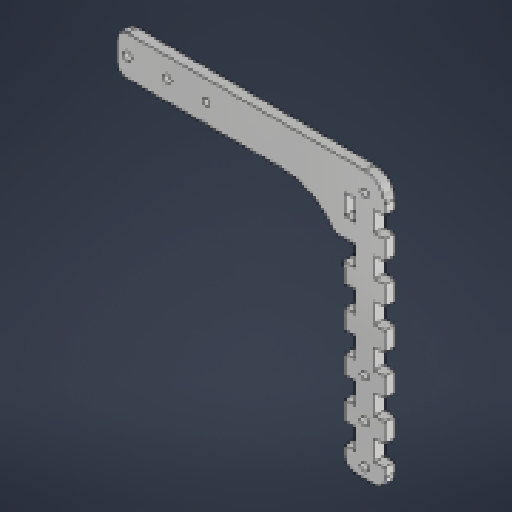
# Autodesk Inventor part: PLATE,CLAMP,MK4i,Swerve,CUSTOM,FRC2026
Saved by Autodesk Inventor 2026.1 (Build 301233020, 233B)
## iProperties
Created: 2021-12-05
Part Number: PLATE,CLAMP,MK4i,Swerve,CUSTOM,FRC2026
Material: Aluminum 7075
Document SubType Name: Modeling
Designer: dave.simone
Density: 2.81 g/cm^3
Appearance: Aluminum - Polished
Mass: 126.09 g
Surface Area: 201.461 cm^2
Volume: 44.872 cm^3
Author: dave.simone
Revision Number: ANY
Autodesk Inventor part; units mm, degrees
ref_plane "XY Plane" through (0, 0, 0) normal (0, 0, 1) x (1, 0, 0)
ref_plane "Work Plane2" through (0, 0, 0) normal (-0.7071068, 0.7071068, 0) x (0, 0, 1)
sketch "Sketch1" plane through (-160.3375, 44.45, 0) normal (0, 0, 1) x (1, 0, 0)
  line L0 (312.7375, -57.15) -> (160.3375, -57.15)
  arc A0 (312.7375, -57.15) -> (319.0875, -50.8) centre (312.7375, -50.8) ccw
  line L1 (319.0875, -38.1) -> (319.0875, -50.8)
  arc A1 (319.0875, -38.1) -> (312.7375, -31.75) centre (312.7375, -38.1) ccw
  line L2 (214.3125, -31.75) -> (312.7375, -31.75)
  line L3 (173.0375, 107.95) -> (173.0375, 9.525)
  arc A2 (173.0375, 107.95) -> (166.6875, 114.3) centre (166.6875, 107.95) ccw
  line L4 (153.9875, 114.3) -> (166.6875, 114.3)
  arc A3 (153.9875, 114.3) -> (147.6375, 107.95) centre (153.9875, 107.95) ccw
  line L5 (147.6375, -44.45) -> (147.6375, 107.95)
  arc A4 (147.6375, -44.45) -> (160.3375, -57.15) centre (160.3375, -44.45) ccw
  line L6 (160.3375, -94.8593) -> (160.3375, 150.6942) construction
  line L7 (109.9282, -44.45) -> (355.4817, -44.45) construction
  arc A5 (173.0375, 9.525) -> (214.3125, -31.75) centre (214.3125, 9.525) ccw
  dimension "d1" = 171.45
  dimension "d2" = 12.7
  dimension "d5" = 25.4
  dimension "d6" = 25.4
  dimension "d8" = 6.35
  dimension "d44" = 41.275
  constraints: 12 end point, 12 point on circle, 12 tangent, 6 centre point, 3 equal radius, 3 perpendicular, 2 parallel, 1 horizontal
  measures "d1" distance between parallel lines of L1 L5
  measures "d2" radius of A4
  measures "d5" distance between parallel lines of L2 L0
  measures "d6" distance between parallel lines of L5 L3
  measures "d8" radius of A0
  measures "d44" radius of A5
extrude "Extrusion1" add sketch "Sketch1" along normal mid plane 6.35
sketch "Sketch2" plane through (-160.3375, 44.45, 3.175) normal (0, 0, 1) x (1, 0, 0)
  line L0 (160.3375, -91.44) -> (160.3375, 148.59) construction
  line L1 (113.3475, -44.45) -> (353.3775, -44.45) construction
  line L2 (319.0875, -50.8) -> (319.0875, -38.1) construction
  point P0 (160.3375, -44.45)
  point P1 (312.7375, -44.45)
  dimension "d13" = 152.4
  constraints: 1 point on line
  measures "d13" distance from line of L0 point (312.738, -44.45)
hole "Hole1" at (152.4, 0, 3.175) direction (0, 0, -1) diameter 5.1054 end through all start extended yes clearance for "Socket Head Cap Screw" size "#10" standard "Ansi Unified Screw Threads"
pattern_linear "Rectangular Pattern1" count 3 spacing 25.4 along (-1, 0, 0) of "Hole1"
sketch "Sketch4" plane through (-160.3375, 44.45, 3.175) normal (0, 0, 1) x (1, 0, 0)
  point P0 (160.3375, -44.45)
  point P1 (160.3375, -44.45)
  constraints: 1 coincident
hole "Hole2" at (0, 0, 3.175) direction (0, 0, -1) diameter 5.1054 end through all start extended yes clearance for "Socket Head Cap Screw" size "#10" standard "Ansi Unified Screw Threads"
mirror "Mirror1" about plane through (0, 0, 0) normal (-0.7071068, 0.7071068, 0) of "Hole1", "Rectangular Pattern1"
sketch "Sketch6" plane through (-160.3375, 44.45, 3.175) normal (0, 0, 1) x (1, 0, 0)
  line L0 (173.0375, 9.525) -> (173.0375, 107.95) construction
  line L1 (147.6375, 107.95) -> (147.6375, -44.45) construction
  line L2 (147.6375, 88.7095) -> (154.1145, 88.7095)
  line L3 (154.1145, 88.7095) -> (154.1145, 101.7905)
  line L4 (154.1145, 101.7905) -> (147.6375, 101.7905)
  line L5 (147.6375, 101.7905) -> (147.6375, 88.7095)
  line L6 (166.6875, 114.3) -> (153.9875, 114.3) construction
  line L7 (166.5605, 88.7095) -> (173.0375, 88.7095)
  line L8 (173.0375, 88.7095) -> (173.0375, 101.7905)
  line L9 (173.0375, 101.7905) -> (166.5605, 101.7905)
  line L10 (166.5605, 101.7905) -> (166.5605, 88.7095)
  point P0 (160.3375, -44.45)
  point P1 (154.1145, 95.25)
  point P2 (173.0375, 95.25)
  dimension "d51" = 6.477
  dimension "d53" = 13.081
  dimension "d54" = 19.05
  dimension "d55" = 6.477
  dimension "d56" = 13.081
  constraints: 16 end point, 4 parallel, 2 collinear, 2 horizontal, 2 midpoint, 2 perpendicular, 1 point on line
  measures "d51" distance of L2.start L2.end
  measures "d53" distance of L2.end L3.end
  measures "d54" distance from line of L6 point (154.114, 95.25)
  measures "d55" distance of L7.start L7.end
  measures "d56" distance of L7.end L8.end
extrude "Extrusion4" cut sketch "Sketch6" against normal through all
pattern_linear "Rectangular Pattern2" count 6 spacing 25.4 along (0, -1, 0) of "Extrusion4"
delete faces "Delete Face1" heal yes whole lump no faces at (12.7, 35.9198, 1.0583)
body "Solid18"
